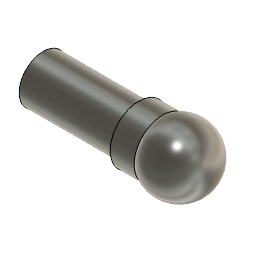
robosoc_leg_piece_V.1 (Autodesk Fusion 360 design; units mm, degrees)
part number: 2025-12-04-11-27-23-377
Autodesk Fusion 360 part; units mm, degrees
sketch "Sketch1" plane through (0, 0, 0) normal (0, 0, 1) x (1, 0, 0)
  line L0 (0, 0) -> (50, 0)
  line L1 (50, 8) -> (50, 10)
  line L2 (40, 10) -> (0, 10)
  line L3 (0, 10) -> (0, 0)
  line L4 (50, 10) -> (40, 10) construction
  line L5 (50, 10) -> (50, 12)
  line L6 (50, 12) -> (40, 12)
  line L7 (40, 12) -> (40, 10)
  line L8 (50, 0) -> (57, 0) construction
  arc A0 (70.8924, 0) -> (50, 12) centre (57, 0) ccw
  arc A1 (69.2066, 0) -> (50, 10) centre (57, 0) ccw
  line L9 (50, 0) -> (70.8924, 0)
  line L10 (0, 0) -> (0, 8) construction
  line L11 (0, 8) -> (50, 8)
  line L12 (50, 8) -> (50, 10)
  dimension "d1" = 50
  dimension "d2" = 10
  dimension "d3" = 10
  dimension "d4" = 10
  dimension "d5" = 2
  dimension "d6" = 7
  dimension "d7" = 8
  dimension "d8" = 50
  constraint horizontal L0
  constraint vertical L1
  constraint horizontal L2
  constraint vertical L3
  constraint coincident L0.start L3.end
  constraint perpendicular L1 L4
  constraint vertical L5
  constraint horizontal L6
  constraint vertical L7
  constraint perpendicular L1 L8
  constraint coincident L8.end A0.centre
  constraint perpendicular L1 L9
  constraint perpendicular L0 L10
  constraint perpendicular L1 L11
  measures "d1" distance of L0.start L0.end
  measures "d2" distance of L0.start L2.end
  measures "d3" distance of L1.end L2.start
  measures "d4" distance of L2.start L1.end
  measures "d5" distance of L2.start L6.end
  measures "d6" distance of L0.end L8.end
  measures "d7" distance of L0.start L10.end
  measures "d8" distance of L10.end L1.start
revolve "Revolve1" add sketch "Sketch1" angle 360 about axis through (0, 0, 0) along (1, 0, 0) contours L1 L2 L3 L5 L6 L7 L11 L12 | L5 A0 A1 L9
